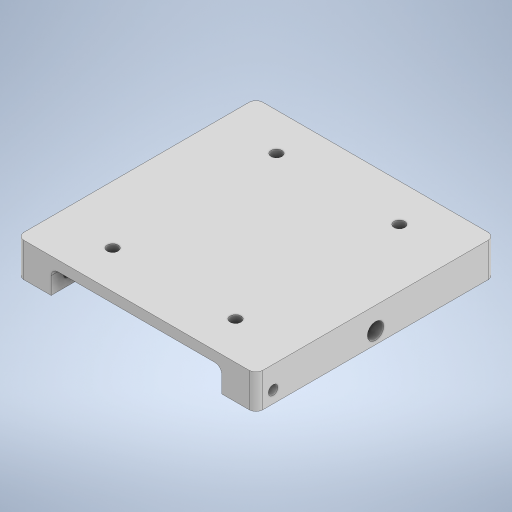
# Autodesk Inventor part: MID-360_mountA
Saved by Autodesk Inventor 2024 (Build 280153000, 153)
## iProperties
Created: 2025-03-31
Part Number: MID-360_mountA
Material: 一般
Document SubType Name: Modeling
Designer: babar
Density: 1 g/cm^3
Appearance: 既定
Author: babar
Autodesk Inventor part; units mm, degrees
ref_plane "YZ Plane" through (0, 0, 0) normal (1, 0, 0) x (0, 1, 0)
ref_plane "XZ Plane" through (0, 0, 0) normal (0, 1, 0) x (-1, 0, 0)
ref_plane "XY Plane" through (0, 0, 0) normal (0, 0, 1) x (1, 0, 0)
sketch "スケッチ1" plane through (0, 0, 0) normal (0, 1, 0) x (-1, 0, 0)
  line L0 (35, -35) -> (-35, -35)
  line L1 (-35, -35) -> (-35, 35)
  line L2 (-35, 35) -> (35, 35)
  line L3 (35, 35) -> (35, -35)
  line L4 (35, -35) -> (-35, 35) construction
  line L5 (-35, -35) -> (35, 35) construction
  point P0 (0, 0)
  dimension "d0" = 70
  dimension "d1" = 70
  constraints: 12 end point, 2 midpoint, 2 parallel, 1 horizontal, 1 perpendicular
  measures "d0" distance of L1.end L2.end
  measures "d1" distance of L0.end L1.end
extrude "押し出し1" add sketch "スケッチ1" along normal blind 10
sketch "スケッチ2" plane through (0, 0, 0) normal (0, -1, 0) x (1, 0, 0)
  line L0 (35, -35) -> (-35, -35) projected
  line L1 (-25, 35) -> (25, 35)
  line L2 (25, 35) -> (25, -35)
  line L3 (25, -35) -> (-25, -35)
  line L4 (-25, -35) -> (-25, 35)
  line L5 (-25, 35) -> (25, -35) construction
  line L6 (25, 35) -> (-25, -35) construction
  point P0 (0, 0)
  dimension "d4" = 50
  constraints: 12 end point, 2 midpoint, 2 parallel, 1 horizontal, 1 perpendicular, 1 point on line
  measures "d4" distance of L2.end L3.end
extrude "押し出し2" cut sketch "スケッチ2" against normal blind 7
sketch "スケッチ3" plane through (-35, 0, -35) normal (-1, 0, 0) x (0, 0, 1)
  line L0 (0, 0) -> (70, 0) projected
  point P0 (35, 0)
  point P1 (35, 3.5)
  point P2 (35, 0)
  dimension "d7" = 3.5
  constraints: 1 midpoint
  measures "d7" distance of point (35, 0) point (35, 3.5)
hole "穴1" at (-35, 3.5, 0) direction (1, 0, 0) diameter 4.8 end through all
sketch "スケッチ4" plane through (0, 10, 0) normal (0, 1, 0) x (1, 0, 0)
  line L0 (35, 35) -> (-35, 35) projected
  line L1 (-35, 35) -> (-35, -35) projected
  point P0 (0, 0)
  point P1 (-18, 24)
  point P2 (18, 24)
  point P3 (-18, -24)
  point P4 (18, -24)
  dimension "d15" = 18
  dimension "d16" = 24
  dimension "d17" = 11
  dimension "d18" = 17
  dimension "d21" = 36
  dimension "d24" = 48
  constraints: 1 horizontal, 1 vertical, 3 other
  measures "d15" horizontal distance of point (0, 0) point (-18, 24)
  measures "d16" vertical distance of point (0, 0) point (-18, 24)
  measures "d17" distance from line of L0 point (-18, 24)
  measures "d18" distance from line of L1 point (-18, 24)
  measures "d21" distance of point (-18, 24) point (18, 24)
  measures "d24" distance of point (-18, 24) point (-18, -24)
hole "穴2" at (-18, 10, -24) at (18, 10, -24) at (-18, 10, 24) at (18, 10, 24) direction (0, -1, 0) diameter 3.2 end through all
sketch "スケッチ5" plane through (-35, 0, -35) normal (-1, 0, 0) x (0, 0, 1)
  line L0 (0, 0) -> (70, 0) projected
  circle A0 centre (35, 3.5) radius 2.4 projected
  point P0 (35, 0)
  point P1 (65, 3.5)
  dimension "d34" = 3.5
  dimension "d35" = 30
  measures "d34" distance from line of L0 point (65, 3.5)
  measures "d35" distance of A0.centre point (65, 3.5)
hole "穴3" at (-35, 3.5, 30) direction (1, 0, 0) diameter 2.8 end through all
fillet "フィレット1" radius 2 6 edges at (-35, 5, 35) (-35, 5, -35) (35, 5, -35) (35, 5, 35) (25, 7, 0) (-25, 7, 0)
